Autodesk Inventor part; units mm, degrees
(part 2 of 2)
  spline S279 degree 2 poles (-4.1824, 60.7666) (-4.1824, 60.8773) (-3.774, 61.341) (-3.774, 61.3687) knots 0 0 0 1 2 2 2
  spline S280 degree 2 poles (-3.774, 61.3687) (-3.774, 61.386) (-3.7948, 61.386) knots 0 0 0 1 1 1
  spline S281 degree 2 poles (-3.7948, 61.386) (-3.8813, 61.386) (-4.1685, 61.1161) knots 0 0 0 1 1 1
  spline S282 degree 2 poles (-4.1685, 61.1161) (-4.4073, 60.8929) (-4.5197, 60.7545) knots 0 0 0 1 1 1
  spline S283 degree 2 poles (-4.5197, 60.7545) (-4.5889, 60.668) (-4.6218, 60.668) knots 0 0 0 1 1 1
  spline S284 degree 2 poles (-4.6218, 60.668) (-4.6772, 60.668) (-4.6772, 60.7199) knots 0 0 0 1 1 1
  spline S285 degree 2 poles (-4.6772, 60.7199) (-4.6772, 60.7718) (-4.2291, 61.2718) (-4.2291, 61.3306) knots 0 0 0 1 2 2 2
  spline S286 degree 2 poles (-4.2291, 61.3306) (-4.2291, 61.3566) (-4.2567, 61.3566) knots 0 0 0 1 1 1
  spline S287 degree 2 poles (-4.2567, 61.3566) (-4.3311, 61.3566) (-4.5958, 61.1074) knots 0 0 0 1 1 1
  spline S288 degree 2 poles (-4.5958, 61.1074) (-4.8225, 60.8946) (-4.9159, 60.7735) knots 0 0 0 1 1 1
  spline S289 degree 2 poles (-4.9159, 60.7735) (-4.9886, 60.6801) (-5.0422, 60.6801) knots 0 0 0 1 1 1
  spline S290 degree 2 poles (-5.0422, 60.6801) (-5.0907, 60.6801) (-5.0907, 60.7234) knots 0 0 0 1 1 1
  spline S291 degree 2 poles (-5.0907, 60.7234) (-5.0907, 60.777) (-4.8917, 61.0244) knots 0 0 0 1 1 1
  line L57 (-4.8917, 61.0244) -> (-4.6616, 61.3099)
  spline S292 degree 2 poles (-3.4834, 60.9725) (-3.8657, 60.6715) (-4.0093, 60.6715) knots 0 0 0 1 1 1
  spline S293 degree 2 poles (-4.0093, 60.6715) (-4.0266, 60.6715) (-4.0266, 60.6905) knots 0 0 0 1 1 1
  spline S294 degree 2 poles (-4.0266, 60.6905) (-4.0266, 60.7182) (-3.992, 60.7234) knots 0 0 0 1 1 1
  spline S295 degree 2 poles (-3.992, 60.7234) (-3.8588, 60.7441) (-3.6201, 60.931) knots 0 0 0 1 1 1
  line L58 (-3.6201, 60.931) -> (-3.4367, 61.0746)
  line L59 (-3.4367, 61.0746) -> (-3.1408, 61.3099)
  spline S296 degree 2 poles (-3.1408, 61.3099) (-2.9384, 61.45) (-2.7931, 61.45) knots 0 0 0 1 1 1
  spline S297 degree 2 poles (-2.7931, 61.45) (-2.6858, 61.45) (-2.6737, 61.3427) knots 0 0 0 1 1 1
  spline S298 degree 2 poles (-2.6737, 61.3427) (-2.6183, 61.3964) (-2.5958, 61.3964) knots 0 0 0 1 1 1
  spline S299 degree 2 poles (-2.5958, 61.3964) (-2.5491, 61.3964) (-2.5491, 61.3566) knots 0 0 0 1 1 1
  spline S300 degree 2 poles (-2.5491, 61.3566) (-2.5491, 61.3064) (-2.9868, 60.796) (-2.9868, 60.7528) knots 0 0 0 1 2 2 2
  spline S301 degree 2 poles (-2.9868, 60.7528) (-2.9868, 60.7234) (-2.8952, 60.7199) (-2.8952, 60.6974) knots 0 0 0 1 2 2 2
  spline S302 degree 2 poles (-2.8952, 60.6974) (-2.8952, 60.668) (-2.9903, 60.668) knots 0 0 0 1 1 1
  spline S303 degree 2 poles (-2.9903, 60.668) (-3.0855, 60.668) (-3.0855, 60.7528) knots 0 0 0 1 1 1
  spline S304 degree 2 poles (-3.0855, 60.7528) (-3.0855, 60.8202) (-3.0093, 60.9431) knots 0 0 0 1 1 1
  line L60 (-3.0093, 60.9431) -> (-3.1858, 60.7926)
  spline S305 degree 2 poles (-3.1858, 60.7926) (-3.3156, 60.6957) (-3.3934, 60.6957) knots 0 0 0 1 1 1
  spline S306 degree 2 poles (-3.3934, 60.6957) (-3.5163, 60.6957) (-3.5163, 60.8202) knots 0 0 0 1 1 1
  spline S307 degree 2 poles (-3.5163, 60.8202) (-3.5163, 60.8894) (-3.4834, 60.9725) knots 0 0 0 1 1 1
  spline S308 degree 2 poles (-2.774, 61.3912) (-2.8588, 61.3912) (-3.3865, 60.8877) (-3.3865, 60.8029) knots 0 0 0 1 2 2 2
  spline S309 degree 2 poles (-3.3865, 60.8029) (-3.3865, 60.7649) (-3.3502, 60.7649) knots 0 0 0 1 1 1
  spline S310 degree 2 poles (-3.3502, 60.7649) (-3.2671, 60.7649) (-2.7325, 61.258) (-2.7325, 61.3445) knots 0 0 0 1 2 2 2
  spline S311 degree 2 poles (-2.7325, 61.3445) (-2.7325, 61.3912) (-2.774, 61.3912) knots 0 0 0 1 1 1
  spline S312 degree 2 poles (-1.9661, 61.104) (-1.5734, 61.4362) (-1.4159, 61.4362) knots 0 0 0 1 1 1
  spline S313 degree 2 poles (-1.4159, 61.4362) (-1.3138, 61.4362) (-1.3138, 61.341) knots 0 0 0 1 1 1
  spline S314 degree 2 poles (-1.3138, 61.341) (-1.3138, 61.2562) (-1.7723, 60.8151) (-1.7723, 60.7701) knots 0 0 0 1 2 2 2
  spline S315 degree 2 poles (-1.7723, 60.7701) (-1.7723, 60.7234) (-1.6685, 60.7164) (-1.6685, 60.6957) knots 0 0 0 1 2 2 2
  spline S316 degree 2 poles (-1.6685, 60.6957) (-1.6685, 60.668) (-1.7723, 60.668) knots 0 0 0 1 1 1
  spline S317 degree 2 poles (-1.7723, 60.668) (-1.8917, 60.668) (-1.8917, 60.7735) knots 0 0 0 1 1 1
  spline S318 degree 2 poles (-1.8917, 60.7735) (-1.8917, 60.8618) (-1.7775, 60.9984) knots 0 0 0 1 1 1
  spline S319 degree 2 poles (-1.7775, 60.9984) (-1.7187, 61.0676) (-1.5664, 61.213) knots 0 0 0 1 1 1
  spline S320 degree 2 poles (-1.5664, 61.213) (-1.4522, 61.322) (-1.4522, 61.3445) knots 0 0 0 1 1 1
  spline S321 degree 2 poles (-1.4522, 61.3445) (-1.4522, 61.3635) (-1.4782, 61.3635) knots 0 0 0 1 1 1
  spline S322 degree 2 poles (-1.4782, 61.3635) (-1.5595, 61.3635) (-1.8311, 61.1455) knots 0 0 0 1 1 1
  spline S323 degree 2 poles (-1.8311, 61.1455) (-2.0595, 60.9656) (-2.1685, 60.8497) knots 0 0 0 1 1 1
  spline S324 degree 2 poles (-2.1685, 60.8497) (-2.3086, 60.7026) (-2.3381, 60.7026) knots 0 0 0 1 1 1
  spline S325 degree 2 poles (-2.3381, 60.7026) (-2.3623, 60.7026) (-2.3986, 60.7476) (-2.3986, 60.7718) knots 0 0 0 1 2 2 2
  spline S326 degree 2 poles (-2.3986, 60.7718) (-2.3986, 60.8047) (-2.2014, 61.0365) knots 0 0 0 1 1 1
  line L61 (-2.2014, 61.0365) -> (-1.9661, 61.3133)
  line L62 (-1.9661, 61.3133) -> (-2.3311, 61.0175)
  line L63 (-2.3311, 61.0175) -> (-2.601, 60.8116)
  spline S327 degree 2 poles (-2.601, 60.8116) (-2.8069, 60.6715) (-2.9159, 60.6715) knots 0 0 0 1 1 1
  spline S328 degree 2 poles (-2.9159, 60.6715) (-2.9349, 60.6715) (-2.9349, 60.6888) knots 0 0 0 1 1 1
  spline S329 degree 2 poles (-2.9349, 60.6888) (-2.9349, 60.7147) (-2.8952, 60.7234) knots 0 0 0 1 1 1
  spline S330 degree 2 poles (-2.8952, 60.7234) (-2.8415, 60.7337) (-2.7671, 60.7666) knots 0 0 0 1 1 1
  spline S331 degree 2 poles (-2.7671, 60.7666) (-2.6633, 60.8116) (-2.3433, 61.0711) knots 0 0 0 1 1 1
  spline S332 degree 2 poles (-2.3433, 61.0711) (-2.0543, 61.3047) (-1.928, 61.4275) knots 0 0 0 1 1 1
  spline S333 degree 2 poles (-1.928, 61.4275) (-1.9055, 61.45) (-1.8606, 61.4794) knots 0 0 0 1 1 1
  spline S334 degree 2 poles (-1.8606, 61.4794) (-1.8381, 61.4881) (-1.8121, 61.4881) knots 0 0 0 1 1 1
  spline S335 degree 2 poles (-1.8121, 61.4881) (-1.7879, 61.4881) (-1.7377, 61.4552) (-1.7377, 61.4327) knots 0 0 0 1 2 2 2
  spline S336 degree 2 poles (-1.7377, 61.4327) (-1.7377, 61.4067) (-1.9661, 61.104) knots 0 0 0 1 1 1
  point P0 (0, 0)
  constraints: 2 other
emboss "Emboss1" sketch "Sketch21" operation cut depth 2 direction (0, 0, 1)
body "Solid1"
